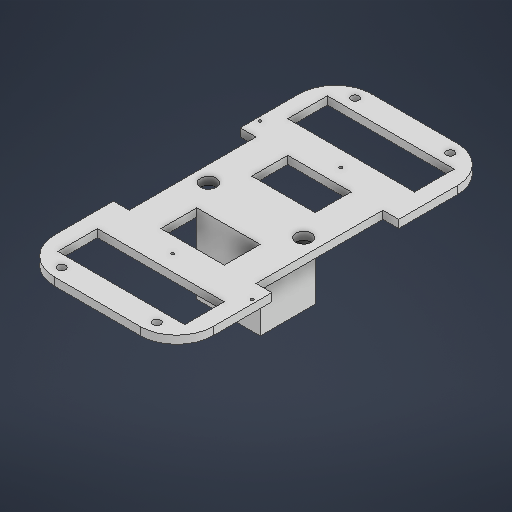
# Autodesk Inventor part: chassis
Saved by Autodesk Inventor 2027 (Build 310192060, 192F)
## iProperties
Created: 2026-07-01
Part Number: chassis
Material: Generic
Document SubType Name: Modeling
Designer: loren
Density: 1 g/cm^3
Appearance: Default
Author: loren
Autodesk Inventor part; units mm, degrees
ref_plane "YZ Plane" through (0, 0, 0) normal (1, 0, 0) x (0, 1, 0)
ref_plane "XZ Plane" through (0, 0, 0) normal (0, 1, 0) x (-1, 0, 0)
ref_plane "XY Plane" through (0, 0, 0) normal (0, 0, 1) x (1, 0, 0)
sketch "Sketch1" plane through (0, 0, 0) normal (0, 1, 0) x (-1, 0, 0)
  line L0 (-25, 50) -> (25, 50)
  line L1 (25, -50) -> (-25, -50)
  line L2 (-25, 50) -> (25, -50) construction
  line L3 (0, 0) -> (0, 10.8306)
  line L4 (0, 10.8306) -> (0, 0)
  line L5 (25, 20) -> (20, 20)
  line L6 (25, -20) -> (20, -20)
  line L7 (20, 20) -> (20, -20)
  line L8 (25, 50) -> (25, 20)
  line L9 (25, -20) -> (25, -50)
  line L10 (20, 42.5) -> (20, 30)
  line L11 (-25, 20) -> (-20, 20)
  line L12 (-25, -20) -> (-20, -20)
  line L13 (-20, 20) -> (-20, -20)
  line L14 (-25, -50) -> (-25, -20)
  line L15 (-25, 20) -> (-25, 50)
  line L16 (-20, 42.5) -> (-20, 30)
  line L17 (10, 8.6721) -> (-10, 8.6721)
  line L18 (0, 0) -> (3.9876, 0)
  line L19 (10, 25) -> (10, 8.6721)
  line L20 (-10, 25) -> (-10, 8.6721)
  circle A0 centre (15, 0) radius 2.5
  circle A1 centre (-15, 0) radius 2.5
  circle A2 centre (15, 10) radius 2.5
  circle A3 centre (15, -10) radius 2.5
  circle A4 centre (-15, 10) radius 2.5
  circle A5 centre (-15, -10) radius 2.5
  circle A6 centre (15, -46.25) radius 1.25
  circle A7 centre (-15, -46.25) radius 1.25
  circle A8 centre (15, 46.25) radius 1.25
  line L21 (20, 42.5) -> (-20, 42.5)
  line L22 (20, 42.5) -> (60, 42.5) construction
  line L23 (20, 30) -> (10, 30)
  line L24 (10, 30) -> (10, 25)
  line L25 (-10, 25) -> (-10, 30)
  line L26 (-10, 30) -> (-20, 30)
  line L27 (0, 42.5) -> (0, 47.5)
  circle A9 centre (-15, 46.25) radius 1.25
  circle A10 centre (15, -46.25) radius 1.25
  circle A11 centre (-15, -46.25) radius 1.25
  line L28 (20, -42.5) -> (20, -30)
  line L29 (-20, -42.5) -> (-20, -30)
  line L30 (10, -8.6721) -> (-10, -8.6721)
  line L31 (10, -25) -> (10, -8.6721)
  line L32 (-10, -25) -> (-10, -8.6721)
  line L33 (20, -42.5) -> (-20, -42.5)
  line L34 (20, -30) -> (10, -30)
  line L35 (10, -30) -> (10, -25)
  line L36 (-10, -25) -> (-10, -30)
  line L37 (-10, -30) -> (-20, -30)
  line L38 (20, 36.25) -> (9.5871, 36.25)
  circle A12 centre (15, 26.25) radius 1.25
  circle A13 centre (-15, 26.25) radius 1.25
  circle A14 centre (15, -26.25) radius 1.25
  circle A15 centre (-15, -26.25) radius 1.25
  line L39 (10, -20) -> (-10, -20)
  line L40 (10, -30) -> (-10, -30)
  line L41 (10, 30) -> (-10, 30)
  line L42 (10, 20) -> (-10, 20)
  point P0 (20, 45)
  point P1 (-20, 45)
  point P2 (20, 0)
  dimension "d0" = 50
  dimension "d1" = 100
  dimension "d2" = 40
  dimension "d7" = 5
  dimension "d16" = 20
  dimension "d22" = 5
  dimension "d23" = 5
  dimension "d25" = 5
  dimension "d28" = 2.5
  dimension "d36" = 180
  dimension "d37" = 2.5
  dimension "d38" = 3.75
  dimension "d39" = 7.5
  dimension "d59" = 10
  dimension "d60" = 5
  constraints: 86 end point, 29 symmetric about line, 16 centre point, 12 point on line, 7 equal length, 7 horizontal, 5 perpendicular, 5 vertical, 4 midpoint, 1 collinear, 13 other
  measures "d0" distance of L1.start L1.end
  measures "d1" distance of L0.end L1.start
  measures "d2" distance of L5.end L6.end
  measures "d7" distance from line of L0 point (20, 45)
  measures "d16" distance of L17.start L17.end
  measures "d22" diameter of A0
  measures "d23" distance of point (20, 0) A0.centre
  measures "d25" diameter of A2
  measures "d28" diameter of A6
  measures "d36" angle of L21 L22
  measures "d37" distance of L10.start point (20, 45)
  measures "d38" distance from line of L0 A8.centre
  measures "d39" vertical distance of L10.start L0.end
  measures "d59" distance from line of L8 A8.centre
  measures "d60" horizontal distance of A8.centre L10.start
extrude "Extrusion2" add sketch "Sketch1" along normal blind 2.5 contours L0 L8 L5 L7 L6 L9 L1 L14 L12 L13 L11 L15 | A2 | A3 | A4 | A5 | A12 | A13 | A14 | A15
extrude "Extrusion3" cut sketch "Sketch1" along normal blind 5 contours A12 | A13 | A14 | A15
extrude "Extrusion5" add sketch "Sketch1" along normal blind 2.5 contours L24 L19 L42 L20 L25 L41 | L40 L36 L32 L39 L31 L35
extrude "Extrusion6" add sketch "Sketch1" along normal blind 2.5 contours A6 | A7 | A8 | A9 | A12 | A13 | A14 | A15
sketch "Sketch2" plane through (0, 2.5, 0) normal (0, 1, 0) x (1, 0, 0)
  line L0 (-25, 50) -> (-25, 20) projected
  line L1 (20, 30) -> (-20, 30) projected
  line L2 (0, 30) -> (0, 26.2998)
  line L3 (0, 0) -> (3.3663, 0)
  line L4 (0, 0) -> (0, -4.2986)
  point P0 (23.75, 25)
  point P1 (-23.75, -25)
  point P2 (1.6831, 25)
  point P3 (-1.25, -25)
  point P4 (23.75, -25)
  point P5 (-23.75, 25)
  constraints: 6 end point, 2 symmetric about line, 2 vertical, 1 horizontal, 1 midpoint
hole "Hole1" at (1.6831, 2.5, -25) at (-23.75, 2.5, -25) at (23.75, 2.5, 25) at (-1.25, 2.5, 25) direction (0, -1, 0) diameter 0.9398 depth 3.65 tip angle 118 thread size "120-102 UNM" class "2B" standard "ANSI Unified Screw Threads"
extrude "Extrusion7" cut sketch "Sketch1" along normal blind 2.5 contours A6 | A7 | A8 | A9
sketch "Sketch3" plane through (0, 0, 0) normal (0, -1, 0) x (1, 0, 0)
  line L0 (-10, -8.6721) -> (-10, -20) projected
  line L1 (10, 8.6721) -> (10, 20) projected
  line L2 (-10, -8.6721) -> (10, -8.6721)
  line L3 (10, -8.6721) -> (10, 8.6721)
  line L4 (10, 8.6721) -> (-10, 8.6721)
  line L5 (-10, 8.6721) -> (-10, -8.6721)
  circle A0 centre (0.0709, -0.0714) radius 10
  line L6 (0.0709, -0.0714) -> (10.0709, -0.0714) construction
  line L7 (7.142, -7.1424) -> (6.0813, -6.0818)
  circle A1 centre (0.0709, -0.0714) radius 7.5
  circle A2 centre (5.3742, 5.2319) radius 1
  line L8 (0.0709, -0.0714) -> (2.8297, -0.0714)
  line L9 (0.0709, -0.0714) -> (0.0709, -2.5376)
  circle A3 centre (5.3742, -5.3747) radius 1
  circle A4 centre (-5.2324, 5.2319) radius 1
  circle A5 centre (-5.2324, -5.3747) radius 1
  point P0 (0, 0)
  dimension "d63" = 2
  constraints: 16 end point, 3 centre point, 3 symmetric about line, 2 horizontal, 2 parallel, 2 perpendicular, 1 point on line, 12 other
  measures "d63" diameter of A2
extrude "Extrusion8" add sketch "Sketch3" along normal blind 22.5 contours L5 L4 A0 L2 | A0 L4 L3 L2 | A0 L3 L2 | L4 L3 A0 | A1 A3 A5 A4 A2 | A2 A1 | A1 A2 | A3 A1 | A1 A3 | A4 A1 | A1 A4 | A5 A1 | A1 A5
sketch "Sketch4" plane through (0, -22.5, 0) normal (0, -1, 0) x (1, 0, 0)
  circle A0 centre (0.0709, -0.0714) radius 10 projected
  circle A1 centre (0.0557, -0.1018) radius 10
  line L0 (0.0557, -0.1018) -> (10.0557, -0.1018) construction
  line L1 (7.1268, -7.1729) -> (6.0661, -6.1122)
  circle A2 centre (0.0557, -0.1018) radius 7.5
  circle A3 centre (5.359, 5.2015) radius 1
  line L2 (0.0557, -0.1018) -> (2.8145, -0.1018)
  line L3 (0.0557, -0.1018) -> (0.0557, -2.568)
  circle A4 centre (5.359, -5.4051) radius 1
  circle A5 centre (-5.2476, 5.2015) radius 1
  circle A6 centre (-5.2476, -5.4051) radius 1
  point P0 (0, 0)
  dimension "d64" = 2
  constraints: 8 end point, 3 centre point, 3 symmetric about line, 1 horizontal, 1 perpendicular, 1 point on line, 12 other
  measures "d64" diameter of A3
extrude "Extrusion9" cut sketch "Sketch4" against normal blind 5 contours A3 A2 | A2 A3 | A4 A2 | A2 A4 | A5 A2 | A2 A5 | A6 A2 | A2 A6
fillet "Fillet1" radius 11.525 4 edges at (25, 1.25, 50) (-25, 1.25, 50) (-25, 1.25, -50) (25, 1.25, -50)
body "Solid2"
